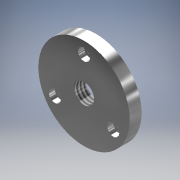
# Autodesk Inventor part: Gripper_Central_Plate_Base
Saved by Autodesk Inventor 2021.3 (Build 253353000, 353)
## iProperties
Created: 2021-04-16
Part Number: Gripper_Central_Plate_Base
Material: Aluminum 6061
Document SubType Name: Modeling
Designer: domin
Density: 2.7 g/cm^3
Appearance: Aluminum - Flat
Mass: 24.7645 g
Surface Area: 44.3301 cm^2
Volume: 9.17205 cm^3
Author: domin
Autodesk Inventor part; units mm, degrees
ref_plane "YZ Plane" through (0, 0, 0) normal (1, 0, 0) x (0, 1, 0)
ref_plane "XZ Plane" through (0, 0, 0) normal (0, 1, 0) x (-1, 0, 0)
ref_plane "XY Plane" through (0, 0, 0) normal (0, 0, 1) x (1, 0, 0)
sketch "Sketch1" plane through (0, 0, 0) normal (0, 0, 1) x (1, 0, 0)
  circle A0 centre (0, 0) radius 23
  dimension "d0" = 46
  constraints: 1 centre point, 1 coincident
  measures "d0" diameter of A0
extrude "Extrusion1" add sketch "Sketch1" along normal mid plane 6
sketch "Sketch2" plane through (0, 0, 3) normal (0, 0, 1) x (1, 0, 0)
  circle A0 centre (0, 17) radius 1.5
  circle A1 centre (-14.7224, -8.5) radius 1.5
  circle A2 centre (14.7224, -8.5) radius 1.5
  point P0 (0, 0)
  dimension "d3" = 3
  dimension "d4" = 17
  dimension "d7" = 360
  constraints: 3 centre point, 1 vertical alignment, 7 other
  measures "d3" diameter of A0
  measures "d4" distance of point (0, 0) A0.centre
hole "Hole1" at (0, 17, 3) at (-14.7224, -8.5, 3) at (14.7224, -8.5, 3) direction (0, 0, -1) diameter 3 end through all counterbore diameter 6 counterbore depth 3
sketch "Sketch3" plane through (0, 0, 3) normal (0, 0, 1) x (1, 0, 0)
  circle A0 centre (0, 0) radius 6
  dimension "d16" = 12
  constraints: 1 centre point, 1 coincident
  measures "d16" diameter of A0
hole "Hole2" at (0, 0, 3) direction (0, 0, -1) diameter 10.106 depth 6 thread size "M12x1.75" class "6H" standard "ISO Metric profile"
equation "\"d9\" = d3"
body "Solid1"
